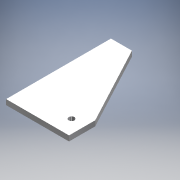
# Autodesk Inventor part: Back Brace
Saved by Autodesk Inventor 2019.4 (Build 234330000, 330)
## iProperties
Created: 2020-01-06
Part Number: Back Brace
Material: Aluminum 6061
Document SubType Name: Modeling
Designer: Mark
Mass: 97.2 g
Surface Area: 161.815 cm^2
Volume: 36 cm^3
Density: 2.7 g/cm^3
Appearance: Aluminum - Flat
Author: Mark
Autodesk Inventor part; units mm, degrees
ref_plane "YZ Plane" through (0, 0, 0) normal (1, 0, 0) x (0, 1, 0)
ref_plane "XZ Plane" through (0, 0, 0) normal (0, 1, 0) x (-1, 0, 0)
ref_plane "XY Plane" through (0, 0, 0) normal (0, 0, 1) x (1, 0, 0)
sketch "Sketch1" plane through (0, 0, 0) normal (0, 1, 0) x (-1, 0, 0)
  line L0 (-30, 50) -> (30, 50)
  line L1 (30, 50) -> (30, -50)
  line L2 (30, -50) -> (-30, -50)
  line L3 (-30, -50) -> (-30, 50)
  line L4 (-30, 50) -> (30, -50) construction
  line L5 (30, 50) -> (-30, -50) construction
  line L6 (-30, 50) -> (30, 50)
  line L7 (30, 50) -> (30, 25)
  line L8 (30, 25) -> (-30, 25)
  line L9 (-30, 25) -> (-30, 50)
  line L10 (30, -50) -> (10, -50)
  line L11 (10, -50) -> (10, 25)
  line L12 (10, 25) -> (30, 25)
  line L13 (30, 25) -> (30, -50)
  line L14 (-30, 25) -> (10, -50)
  point P0 (0, 0)
  dimension "d0" = 60
  dimension "d1" = 100
  dimension "d2" = 25
  dimension "d3" = 20
  constraints: 30 end point, 6 parallel, 3 horizontal, 3 perpendicular, 2 midpoint, 2 point on line
  measures "d0" distance of L1.end L2.end
  measures "d1" distance of L0.end L1.end
  measures "d2" distance of L6.end L7.end
  measures "d3" distance of L11.end L12.end
extrude "Extrusion1" add sketch "Sketch1" along normal blind 5 contours L0 L1 L8 L3 | L8 L11 L14 | L1 L2 L11 L8
sketch "Sketch2" plane through (0, 5, 0) normal (0, 1, 0) x (1, 0, 0)
  circle A0 centre (17.5, -35) radius 2.75
  line L0 (-30, 50) -> (-30, -50) projected
  line L1 (-30, -50) -> (30, -50) projected
  circle A1 centre (-20, -9) radius 2.75
  circle A2 centre (-20, 41) radius 2.75
  point P0 (0, 0)
  dimension "d6" = 5.5
  dimension "d7" = 47.5
  dimension "d8" = 15
  dimension "d11" = 5.5
  dimension "d12" = 10
  dimension "d13" = 41
  dimension "d14" = 5.5
  dimension "d15" = 10
  dimension "d16" = 50
  constraints: 3 centre point
  measures "d6" diameter of A0
  measures "d7" distance from line of L0 A0.centre
  measures "d8" distance from line of L1 A0.centre
  measures "d11" diameter of A1
  measures "d12" distance from line of L0 A1.centre
  measures "d13" distance from line of L1 A1.centre
  measures "d14" diameter of A2
  measures "d15" distance from line of A2.centre L0
  measures "d16" distance of A1.centre A2.centre
extrude "Extrusion2" cut sketch "Sketch2" against normal blind 5
fillet "Fillet1" radius 2 2 edges at (30, 2.5, 25) (-10, 2.5, -50)
body "Solid1"
